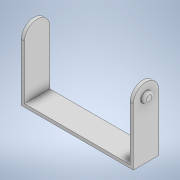
# Autodesk Inventor part: box bot
Saved by Autodesk Inventor 2021 (Build 250183000, 183)
## iProperties
Created: 2021-06-29
Part Number: box bot
Material: Generic
Document SubType Name: Modeling
Designer: newic
Density: 1 g/cm^3
Appearance: Default
Author: newic
Autodesk Inventor part; units mm, degrees
ref_plane "YZ Plane" through (0, 0, 0) normal (1, 0, 0) x (0, 1, 0)
ref_plane "XZ Plane" through (0, 0, 0) normal (0, 1, 0) x (-1, 0, 0)
ref_plane "XY Plane" through (0, 0, 0) normal (0, 0, 1) x (1, 0, 0)
sketch "Sketch1" plane through (0, 0, 0) normal (1, 0, 0) x (0, 1, 0)
  arc A0 (0, -12.7) -> (0, 12.7) centre (0, 0) ccw
  line L0 (0, -12.7) -> (-57.15, -12.7)
  line L1 (-57.15, -12.7) -> (-57.15, 12.7)
  line L2 (-57.15, 12.7) -> (0, 12.7)
  dimension "d0" = 25.4
  dimension "d1" = 57.15
  constraints: 6 end point, 2 point on circle, 2 tangent, 1 centre point, 1 coincident, 1 horizontal, 1 perpendicular
  measures "d0" diameter of A0
  measures "d1" distance of L0.start L0.end
extrude "Extrusion1" add sketch "Sketch1" against normal blind 111.76
sketch "Sketch2" plane through (0, -57.15, 12.7) normal (0, 0, 1) x (1, 0, 0)
  line L0 (0, 57.15) -> (0, 0) projected
  line L1 (0, 57.15) -> (-111.76, 57.15) projected
  line L2 (-111.76, 0) -> (-111.76, 57.15) projected
  line L3 (0, 0) -> (-111.76, 0) projected
  line L4 (-108.585, 3.175) -> (-108.585, 53.975)
  line L5 (-108.585, 53.975) -> (-3.175, 53.975)
  line L6 (-3.175, 53.975) -> (-3.175, 3.175)
  line L7 (-3.175, 3.175) -> (-108.585, 3.175)
  line L8 (-108.585, 53.975) -> (-108.585, 116.1509)
  line L9 (-108.585, 116.1509) -> (-5.0285, 113.469)
  line L10 (-3.175, 53.975) -> (-3.175, 108.1053)
  line L11 (-3.175, 108.1053) -> (-18.8552, 122.8908)
  point P0 (-8.9715, 113.5711)
  dimension "d4" = 3.175
  constraints: 16 end point, 2 vertical, 3 other
  measures "d4" distance between parallel lines of L3 L7
extrude "Extrusion2" cut sketch "Sketch2" against normal blind 111.76 contours L10 L5 L8 L1 | L1 L8 L9 L11 L10 | L6 L7 L4 L5
sketch "Sketch3" plane through (0, 0, 0) normal (1, 0, 0) x (0, 0, -1)
  circle A0 centre (0, 0) radius 5.3975
  dimension "d7" = 10.795
  constraints: 1 centre point, 1 coincident
  measures "d7" diameter of A0
sketch "Sketch4" plane through (-111.76, 0, 0) normal (-1, 0, 0) x (0, 0, 1)
  circle A0 centre (0, 0) radius 5.3975
  dimension "d8" = 10.795
  constraints: 1 centre point, 1 coincident
  measures "d8" diameter of A0
extrude "Extrusion3" add sketch "Sketch4" along normal blind 3.175
fillet "Fillet1" radius 2.54 1 edges at (-114.935, 0, -5.3975)
extrude "Extrusion4" add sketch "Sketch3" along normal blind 3.175
fillet "Fillet2" radius 2.54 1 edges at (3.175, 0, 5.3975)
body "Solid1"
